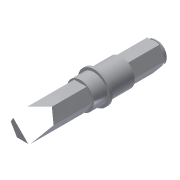
# Autodesk Inventor part: Module Top Shaft
Saved by Autodesk Inventor 2014 SP1 (Build 180222100, 222)
## iProperties
Created: 2014-05-05
Part Number: Module Top Shaft
Material: Aluminum 6061
Document SubType Name: Modeling
Designer: Rauhul Varma
Mass: 3.31629 g
Surface Area: 6.9078 cm^2
Volume: 1.22372 cm^3
Density: 2.71 g/cm^3
Appearance: Aluminum - Flat
Author: Rauhul Varma
Autodesk Inventor part; units mm, degrees
ref_plane "YZ Plane" through (0, 0, 0) normal (1, 0, 0) x (0, 1, 0)
ref_plane "XZ Plane" through (0, 0, 0) normal (0, 1, 0) x (-1, 0, 0)
ref_plane "XY Plane" through (0, 0, 0) normal (0, 0, 1) x (1, 0, 0)
sketch "Sketch1" plane through (0, 0, 0) normal (0, 0, 1) x (1, 0, 0)
  circle A0 centre (0, 0) radius 4.7625
  dimension "d0" = 9.525
  constraints: 1 centre point, 1 coincident
  measures "d0" diameter of A0
extrude "Extrusion1" add sketch "Sketch1" along normal blind 0.7937
sketch "Sketch2" plane through (0, 0, 0.7937) normal (0, 0, 1) x (1, 0, 0)
  circle A0 centre (0, 0) radius 4.7625 projected
  circle A1 centre (0, 0) radius 4.445
  dimension "d3" = 8.89
  constraints: 1 centre point, 1 coincident
  measures "d3" diameter of A1
extrude "Extrusion2" add sketch "Sketch2" along normal blind 0.7366 contours A1
sketch "Sketch3" plane through (0, 0, 1.5304) normal (0, 0, 1) x (1, 0, 0)
  circle A0 centre (0, 0) radius 4.445 projected
  line L0 (5.4993, 0) -> (2.7496, -4.7625)
  line L1 (2.7496, -4.7625) -> (-2.7496, -4.7625)
  line L2 (-2.7496, -4.7625) -> (-5.4993, 0)
  line L3 (-5.4993, 0) -> (-2.7496, 4.7625)
  line L4 (-2.7496, 4.7625) -> (2.7496, 4.7625)
  line L5 (2.7496, 4.7625) -> (5.4993, 0)
  dimension "d6" = 9.525
  constraints: 12 end point, 1 coincident, 1 horizontal, 13 other
  measures "d6" distance between parallel lines of L1 L4
extrude "Extrusion3" add sketch "Sketch3" along normal blind 14.273 contours A0 | L0 L1 L2 L3 L4 L5
sketch "Sketch4" plane through (0, 0, 15.8034) normal (0, 0, 1) x (1, 0, 0)
  circle A0 centre (0, 0) radius 6
  dimension "d9" = 12
  constraints: 1 centre point, 1 coincident
  measures "d9" diameter of A0
extrude "Extrusion4" add sketch "Sketch4" along normal blind 10.9219
sketch "Sketch5" plane through (0, 0, 26.7252) normal (0, 0, 1) x (1, 0, 0)
  circle A0 centre (0, 0) radius 6 projected
  circle A1 centre (0, 0) radius 7.1437
  dimension "d12" = 14.2875
  constraints: 1 centre point, 1 coincident
  measures "d12" diameter of A1
extrude "Extrusion5" add sketch "Sketch5" along normal blind 1.1906 contours A0 | A1
sketch "Sketch6" plane through (0, 0, 27.9159) normal (0, 0, 1) x (1, 0, 0)
  circle A0 centre (0, 0) radius 7.1437 projected
  circle A1 centre (0, 0) radius 6
  dimension "d15" = 12
  constraints: 1 centre point, 1 coincident
  measures "d15" diameter of A1
extrude "Extrusion6" add sketch "Sketch6" along normal blind 6 contours A1
sketch "Sketch7" plane through (0, 0, 33.9159) normal (0, 0, 1) x (1, 0, 0)
  circle A0 centre (0, 0) radius 6 projected
  line L0 (2.7496, 4.7625) -> (5.4993, 0)
  line L1 (5.4993, 0) -> (2.7496, -4.7625)
  line L2 (2.7496, -4.7625) -> (-2.7496, -4.7625)
  line L3 (-2.7496, -4.7625) -> (-5.4993, 0)
  line L4 (-5.4993, 0) -> (-2.7496, 4.7625)
  line L5 (-2.7496, 4.7625) -> (2.7496, 4.7625)
  dimension "d18" = 9.525
  constraints: 12 end point, 1 coincident, 1 horizontal, 13 other
  measures "d18" distance between parallel lines of L2 L5
extrude "Extrusion7" add sketch "Sketch7" along normal blind 25.4 contours L0 L1 L2 L3 L4 L5
chamfer "Chamfer1" distance 0.3969 angle 45 1 edges at (-4.7625, 0, 0)
body "Solid1"
